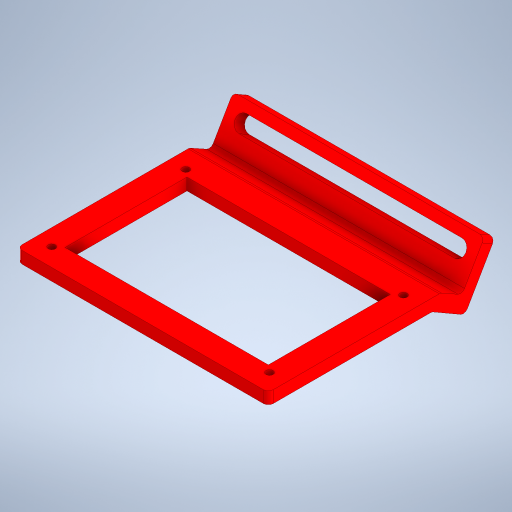
# Autodesk Inventor part: screen mount
Saved by Autodesk Inventor 2023 (Build 270158000, 158)
## iProperties
Created: 2023-03-29
Part Number: screen mount
Material: Generic
Document SubType Name: Modeling
Designer: Steven
Density: 1 g/cm^3
Appearance: Default
Author: Steven
Autodesk Inventor part; units mm, degrees
ref_plane "YZ Plane" through (0, 0, 0) normal (1, 0, 0) x (0, 1, 0)
ref_plane "XZ Plane" through (0, 0, 0) normal (0, 1, 0) x (-1, 0, 0)
ref_plane "XY Plane" through (0, 0, 0) normal (0, 0, 1) x (1, 0, 0)
sketch "Sketch1" plane through (0, 0, 0) normal (0, 1, 0) x (-1, 0, 0)
  line L0 (0, 0) -> (-85, 0)
  line L1 (-85, 0) -> (-85, -51)
  line L2 (-85, -51) -> (0, -51)
  line L3 (0, -51) -> (0, 0)
  line L4 (10, -71) -> (-95, -71)
  line L5 (-95, -71) -> (-95, 10)
  line L6 (10, 10) -> (10, -71)
  line L7 (10, 10) -> (-95, 10)
  circle A0 centre (-88, -53.5) radius 1.5
  line L8 (-42.5, -71) -> (-42.5, 10) construction
  circle A1 centre (3, -53.5) radius 1.5
  line L9 (0, -25.5) -> (-85, -25.5) construction
  circle A2 centre (-88, 2.5) radius 1.5
  circle A3 centre (3, 2.5) radius 1.5
  dimension "d0" = 85
  dimension "d1" = 51
  dimension "d2" = 20
  dimension "d3" = 10
  dimension "d4" = 10
  dimension "d13" = 2.5
  dimension "d14" = 3
  dimension "d15" = 3
  dimension "d34" = 10
  constraints: 20 end point, 4 centre point, 4 midpoint, 3 parallel, 3 symmetric about line, 2 horizontal, 1 perpendicular, 3 other
  measures "d0" distance of L1.end L2.end
  measures "d1" distance of L0.end L1.end
  measures "d2" distance between parallel lines of L2 L4
  measures "d3" distance between parallel lines of L7 L0
  measures "d4" distance between parallel lines of L6 L3
  measures "d13" distance from line of L2 A0.centre
  measures "d14" distance from line of A0.centre L1
  measures "d15" diameter of A0
  measures "d34" distance between parallel lines of L5 L1
extrude "Extrusion1" add sketch "Sketch1" along normal blind 5
sketch "Sketch2" plane through (95, 0, 10) normal (1, 0, 0) x (0, 0, -1)
  line L0 (68, -22.5167) -> (68, 0) construction
  line L1 (82.1908, -7.9375) -> (94.6908, 13.7132)
  line L2 (0, 0) -> (81, 0) construction
  line L3 (81, 5) -> (81, 0)
  line L4 (94.6908, 13.7132) -> (90.3607, 16.2132)
  line L5 (90.3607, 16.2132) -> (81, 0)
  line L6 (68.4427, 0) -> (82.1908, -7.9375)
  line L7 (81, 0) -> (68.4427, 0)
  point P0 (10, 0)
  dimension "d16" = 30
  dimension "d18" = 13
  dimension "d26" = 5
  dimension "d33" = 45
  dimension "d37" = 25
  constraints: 14 end point, 4 perpendicular, 2 point on line, 1 collinear, 1 vertical
  measures "d16" angle of L0 L1
  measures "d18" distance between parallel lines of L3 L0
  measures "d26" distance of L1.end L4.end
  measures "d33" distance of L0.start L1.end
  measures "d37" distance of L1.start L1.end
extrude "Extrusion2" add sketch "Sketch2" against normal blind 105
sketch "Sketch3" plane through (95, -32.5167, -58) normal (0, -0.5, -0.866) x (-1, 0, 0)
  line L0 (7.5, 46.3816) -> (97.5, 46.3816) construction
  line L1 (7.5, 43.1316) -> (97.5, 43.1316)
  line L2 (97.5, 49.6316) -> (7.5, 49.6316)
  arc A0 (7.5, 49.6316) -> (7.5, 43.1316) centre (7.5, 46.3816) ccw
  arc A1 (97.5, 43.1316) -> (97.5, 49.6316) centre (97.5, 46.3816) ccw
  line L3 (0, 53.3816) -> (105, 53.3816) construction
  point P0 (95, -0.8397)
  point P1 (52.5, 46.3816)
  point P2 (52.5, 53.3816)
  point P3 (52.5, 53.3816)
  dimension "d21" = 6.5
  dimension "d22" = 90
  dimension "d23" = 7
  constraints: 8 end point, 4 point on circle, 4 tangent, 3 midpoint, 2 centre point, 1 horizontal, 1 parallel, 1 vertical alignment
  measures "d21" distance between parallel lines of L1 L2
  measures "d22" distance of L2.start L2.end
  measures "d23" distance of point (52.5, 53.382) point (52.5, 46.382)
extrude "Extrusion3" cut sketch "Sketch3" against normal through all
sketch "Sketch4" plane through (95, 0, 10) normal (1, 0, 0) x (0, 0, -1)
  line L0 (81, 0) -> (81, 5) projected
  line L1 (81, 0) -> (72, 5)
  line L2 (72, 5) -> (81, 5)
  line L3 (81, 5) -> (81, 0)
  point P0 (10, 0)
  dimension "d28" = 9
  constraints: 6 end point, 2 perpendicular
  measures "d28" horizontal distance of L0.start L1.end
extrude "Extrusion4" cut sketch "Sketch4" against normal through all
fillet "Fillet3" radius 2 3 edges at (-10, 14.9632, -82.5257) (95, 14.9632, -82.5257) (42.5, 0, -71)
fillet "Fillet4" radius 2 1 edges at (42.5, -7.9375, -72.1908)
fillet "Fillet5" radius 2 2 edges at (42.5, 5, -62) (42.5, 0, -58.4427)
fillet "Fillet6" radius 2 2 edges at (-10, 2.5, 10) (95, 2.5, 10)
equation "\"d34\" = d4"
body "Solid1"
